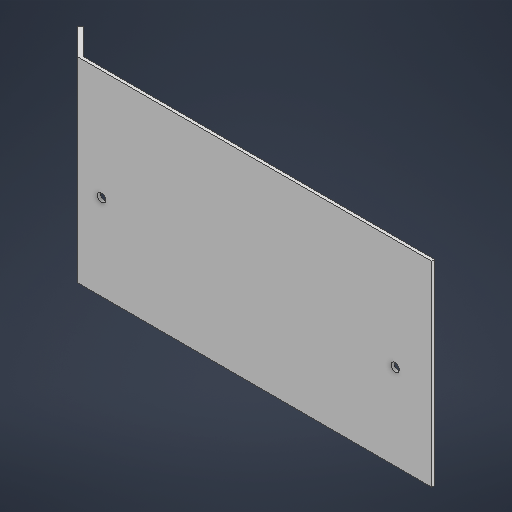
# Autodesk Inventor part: frontwing
Saved by Autodesk Inventor 2026.1 (Build 301233000, 233)
## iProperties
Created: 2026-03-09
Part Number: frontwing
Material: Generic
Document SubType Name: Modeling
Designer: roejo
Density: 1 g/cm^3
Appearance: Default
Author: roejo
Autodesk Inventor part; units mm, degrees
ref_plane "YZ Plane" through (0, 0, 0) normal (1, 0, 0) x (0, 1, 0)
ref_plane "XZ Plane" through (0, 0, 0) normal (0, 1, 0) x (-1, 0, 0)
ref_plane "XY Plane" through (0, 0, 0) normal (0, 0, 1) x (1, 0, 0)
sketch "Sketch1" plane through (0, 0, 0) normal (0, 0, 1) x (1, 0, 0)
  line L0 (0, 0) -> (-184.15, 0)
  line L1 (-184.15, 0) -> (-184.15, 101.6)
  line L2 (-184.15, 101.6) -> (0, 101.6)
  line L3 (0, 101.6) -> (0, 0)
  dimension "d0" = 184.15
  dimension "d1" = 101.6
  constraints: 8 end point, 2 parallel, 1 horizontal, 1 perpendicular
  measures "d0" distance of L1.end L2.end
  measures "d1" distance of L0.end L1.end
extrude "Extrusion1" add sketch "Sketch1" along normal blind 1.5875
chamfer "Chamfer1" distance 1.5875 angle 45 1 edges at (-184.15, 50.8, 0)
sketch "Sketch2" plane through (-184.15, 0, 1.5875) normal (-0.7071068, 0, -0.7071068) x (-0.7071068, 0, 0.7071068)
  line L0 (0, 101.6) -> (0, 0) projected
  line L1 (-2.2451, 101.6) -> (-2.2451, 0) projected
  line L2 (0, 101.6) -> (-2.2451, 101.6) projected
  line L3 (-2.2451, 0) -> (0, 0) projected
  point P0 (-131.3362, 0)
extrude "Extrusion2" add sketch "Sketch2" along normal blind 19.05
sketch "Sketch3" plane through (0, 0, 1.5875) normal (0, 0, 1) x (1, 0, 0)
  circle A0 centre (-19.05, 44.45) radius 2.1844
  line L0 (-184.15, 0) -> (0, 0) projected
  line L1 (-184.15, 101.6) -> (-184.15, 0) projected
  circle A1 centre (-171.45, 44.45) radius 2.1844
  point P0 (-231.8428, 57.2075)
  point P1 (-184.15, 46.6344)
  point P2 (-184.15, 42.2656)
  dimension "d9" = 4.3688
  dimension "d10" = 44.45
  dimension "d11" = 165.1
  dimension "d17" = 4.3688
  dimension "d18" = 152.4
  constraints: 2 centre point
  measures "d9" diameter of A0
  measures "d10" distance from line of L0 A0.centre
  measures "d11" distance from line of A0.centre L1
  measures "d17" diameter of A1
  measures "d18" distance of A0.centre A1.centre
extrude "Extrusion3" cut sketch "Sketch3" against normal blind 19.05
body "Solid1"
